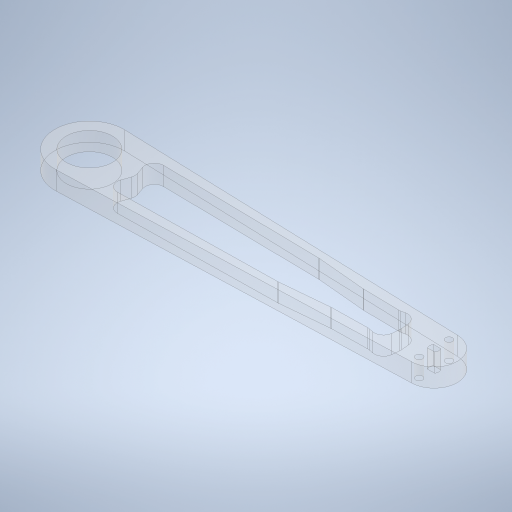
# Autodesk Inventor part: Part2
Saved by Autodesk Inventor 2024 (Build 280153000, 153)
## iProperties
Created: 2024-08-06
Part Number: Part2
Material: Polycarbonate, Clear
Document SubType Name: Modeling
Designer: David Ricaurte
Mass: 37.8047 g
Surface Area: 115.022 cm^2
Volume: 31.5039 cm^3
Density: 1.2 g/cm^3
Appearance: Polycarbonate - Clear
Author: David Ricaurte
Autodesk Inventor part; units mm, degrees
ref_plane "YZ Plane" through (0, 0, 0) normal (1, 0, 0) x (0, 1, 0)
ref_plane "XZ Plane" through (0, 0, 0) normal (0, 1, 0) x (-1, 0, 0)
ref_plane "XY Plane" through (0, 0, 0) normal (0, 0, 1) x (1, 0, 0)
sketch "Sketch1" plane through (0, 0, 0) normal (0, 1, 0) x (-1, 0, 0)
  line L0 (0, 8.5) -> (0, 6.3)
  line L1 (0, -6.3) -> (0, -8.5)
  line L2 (0, 0) -> (150, 0)
  circle A0 centre (150, 0) radius 10
  circle A1 centre (150, 0) radius 15
  circle A2 centre (0, 0) radius 2
  circle A3 centre (0, 0) radius 1.3
  line L3 (0, 1.3) -> (1.5199, 1.3)
  line L4 (0, 1.3) -> (-1.5199, 1.3)
  line L5 (0, -1.3) -> (1.5199, -1.3)
  line L6 (0, -1.3) -> (-1.5199, -1.3)
  circle A4 centre (0, 0) radius 10
  line L7 (0, 10) -> (149.4994, 14.9916)
  line L8 (0, -10) -> (149.4994, -14.9916)
  dimension "d8" = 30
  dimension "d13" = 20
  dimension "d6" = 150
  dimension "d7" = 20
  dimension "d11" = 4
  dimension "d12" = 2.6
  constraints: 18 end point, 6 point on circle, 5 coincident, 3 centre point, 2 horizontal, 2 point on line, 2 symmetric about line, 2 tangent, 2 vertical, 1 parallel, 7 other
  measures "d6" distance of L2.start L2.end
  measures "d7" diameter of A0
  measures "d11" diameter of A2
  measures "d12" diameter of A3
extrude "Extrusion2" add sketch "Sketch1" against normal blind 8 contours L4 A2 L3 | L5 A2 L6 | A4 L7 A1 L2 | A4 | L2 A1 L8 A4 | A1
sketch "Sketch3" plane through (0, 0, 0) normal (0, 1, 0) x (1, 0, 0)
  line L0 (-14.4626, 0) -> (-15.2355, -8.0607)
  line L1 (-15.2355, -8.0607) -> (-21.6951, -6.6804)
  line L2 (-21.6951, -6.6804) -> (-37.7613, -6.9565)
  line L3 (-37.7613, -6.9565) -> (-58.9067, -8.8888)
  line L4 (-58.9067, -8.8888) -> (-133.4402, -10.1695)
  line L5 (-133.4402, -10.1695) -> (-129.907, 0)
  line L6 (-129.907, 0) -> (-14.4626, 0)
  line L7 (-14.4626, 0) -> (-15.2355, 8.0607)
  line L8 (-15.2355, 8.0607) -> (-21.6951, 6.6804)
  line L9 (-21.6951, 6.6804) -> (-37.7613, 6.9565)
  line L10 (-37.7613, 6.9565) -> (-58.9067, 8.8888)
  line L11 (-58.9067, 8.8888) -> (-133.4402, 10.1695)
  line L12 (-133.4402, 10.1695) -> (-129.907, 0)
  point P0 (0, 0)
  constraints: 26 end point, 5 symmetric about line, 1 horizontal, 1 parallel
extrude "Extrusion3" cut sketch "Sketch3" against normal through all
fillet "Fillet1" radius 4 12 edges at (-15.2355, -4, -8.0607) (-14.4626, -4, 0) (-15.2355, -4, 8.0607) (-21.6951, -4, 6.6804) (-37.7613, -4, 6.9565) (-21.6951, -4, -6.6804) (-37.7613, -4, -6.9565) (-58.9067, -4, -8.8888) (-133.4402, -4, -10.1695) (-129.907, -4, 0) (-133.4402, -4, 10.1695) (-58.9067, -4, 8.8888)
sketch "Sketch4" plane through (0, 0, 0) normal (0, 1, 0) x (1, 0, 0)
  circle A0 centre (0, 0) radius 6.5
  circle A1 centre (0, 6.5) radius 1.5
  circle A2 centre (0, -6.5) radius 1.5
  dimension "d19" = 13
  dimension "d20" = 3
  dimension "d21" = 3
  constraints: 3 centre point, 2 point on circle, 1 coincident
  measures "d19" diameter of A0
  measures "d20" diameter of A1
  measures "d21" diameter of A2
extrude "Extrusion4" cut sketch "Sketch4" against normal through all contours A1 A0 | A0 A1 | A2 A0 | A0 A2
body "Solid2"
